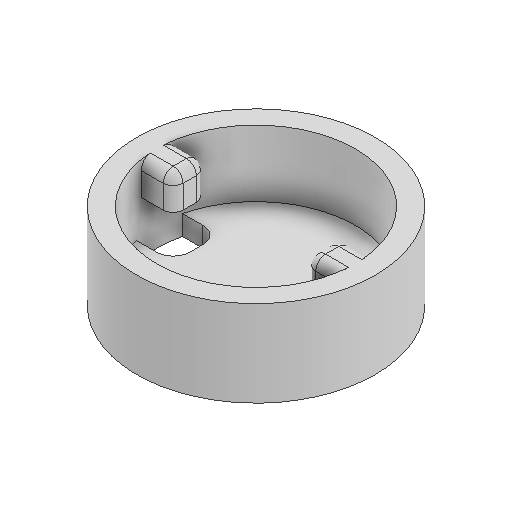
# Autodesk Inventor part: Tapa
Saved by Autodesk Inventor 2025.2 (Build 292293000, 293)
## iProperties
Created: 2025-05-04
Part Number: Tapa
Material: Genérico
Document SubType Name: Modeling
Designer: acer
Density: 1 g/cm^3
Appearance: Valor por defecto
Author: acer
Autodesk Inventor part; units mm, degrees
ref_plane "YZ Plane" through (0, 0, 0) normal (1, 0, 0) x (0, 1, 0)
ref_plane "XZ Plane" through (0, 0, 0) normal (0, 1, 0) x (-1, 0, 0)
ref_plane "XY Plane" through (0, 0, 0) normal (0, 0, 1) x (1, 0, 0)
sketch "Sketch5" plane through (0, 0, 0) normal (0, 1, 0) x (-1, 0, 0)
  circle A0 centre (0, 0) radius 15
  circle A1 centre (0, 0) radius 18
  dimension "d18" = 30
  dimension "d19" = 36
  constraints: 2 centre point, 2 coincident
  measures "d18" diameter of A0
  measures "d19" diameter of A1
extrude "Extrusion4" add sketch "Sketch5" along normal blind 5
sketch "Sketch6" plane through (0, 0, 0) normal (0, -1, 0) x (1, 0, 0)
  circle A0 centre (0, 0) radius 15 projected
  circle A1 centre (0, 0) radius 18 projected
extrude "Extrusion5" add sketch "Sketch6" along normal blind 3 contours A0 | A1
sketch "Sketch7" plane through (0, 5, 0) normal (0, 1, 0) x (1, 0, 0)
  circle A0 centre (0, 0) radius 15 projected
  circle A1 centre (0, 0) radius 18 projected
  line L0 (-17.8255, 2.5) -> (17.8255, 2.5)
  line L1 (-17.8255, -2.5) -> (17.8255, -2.5)
  circle A2 centre (0, 0) radius 10
  line L2 (-10, 2.5) -> (-10, -2.5)
  line L3 (10, 2.5) -> (10, -2.5)
  point P0 (0, 2.5)
  point P1 (-14.7902, 2.5)
  point P2 (14.7902, 2.5)
  point P3 (14.7902, -2.5)
  point P4 (-14.7902, -2.5)
  dimension "d24" = 2.5
  dimension "d25" = 20
  constraints: 8 end point, 4 point on circle, 4 point on line, 1 centre point, 1 coincident, 1 horizontal, 1 midpoint, 1 parallel, 1 perpendicular
  measures "d24" distance of point (0, 2.5) point (0, 0)
  measures "d25" diameter of A2
extrude "Extrusion6" add sketch "Sketch7" along normal blind 5 contours A0 L1 L3 L0 | A0 L0 A1 L1 | A0 L0 A1 | L1 A1 A0 | L0 L2 L1 A0 | A0 L1 A1 L0
fillet "Fillet1" radius 1.5 10 edges at (-10, 7.5, 2.5) (-10, 10, 0) (10, 7.5, 2.5) (10, 10, 0) (10, 7.5, -2.5) (-10, 7.5, -2.5) (12.3951, 10, 2.5) (12.3951, 10, -2.5) (-12.3951, 10, 2.5) (-12.3951, 10, -2.5)
sketch "Sketch8" plane through (0, 0, 0) normal (0, 1, 0) x (1, 0, 0)
  arc A0 (-10, 1) -> (-11.5, 2.5) centre (-11.5, 1) ccw projected
  line L0 (-11.5, 2.5) -> (-14.7902, 2.5) projected
  line L1 (-10, -1) -> (-10, 1) projected
  arc A1 (-11.5, -2.5) -> (-10, -1) centre (-11.5, -1) ccw projected
  line L2 (-14.7902, -2.5) -> (-11.5, -2.5) projected
  line L3 (11.5, -2.5) -> (14.7902, -2.5) projected
  arc A2 (10, -1) -> (11.5, -2.5) centre (11.5, -1) ccw projected
  line L4 (10, 1) -> (10, -1) projected
  arc A3 (11.5, 2.5) -> (10, 1) centre (11.5, 1) ccw projected
  line L5 (14.7902, 2.5) -> (11.5, 2.5) projected
  arc A4 (14.9666, 1) -> (-14.9666, 1) centre (0, 0) ccw projected
  line L6 (-14.7902, -3.5) -> (-11.5, -3.5)
  arc A5 (-11.5, -3.5) -> (-9, -1) centre (-11.5, -1) ccw
  line L7 (-9, -1) -> (-9, 1)
  arc A6 (-9, 1) -> (-11.5, 3.5) centre (-11.5, 1) ccw
  line L8 (-11.5, 3.5) -> (-14.7902, 3.5)
  line L9 (14.7902, -3.5) -> (11.5, -3.5)
  arc A7 (9, -1) -> (11.5, -3.5) centre (11.5, -1) ccw
  line L10 (9, -1) -> (9, 1)
  arc A8 (11.5, 3.5) -> (9, 1) centre (11.5, 1) ccw
  line L11 (11.5, 3.5) -> (14.7902, 3.5)
  circle A9 centre (0, 0) radius 15 projected
  point P0 (14.586, 3.5)
  point P1 (14.586, -3.5)
  point P2 (-14.586, -3.5)
  point P3 (-14.586, 3.5)
  dimension "d29" = 1
  dimension "d30" = 1
  constraints: 12 end point, 8 point on circle, 4 centre point, 8 other
  measures "d29" distance between parallel lines of L2 L6
  measures "d30" radial gap between concentric circles of A3 A8
extrude "Extrusion7" cut sketch "Sketch8" against normal through all contours L1 A1 L2 A9 A4 L0 A0 | A0 L0 A4 L8 A6 L7 A5 L6 A9 L2 A1 L1 | A4 L5 A3 L4 A2 L3 A9 L9 A7 L10 A8 L11 | A4 A9 L3 A2 L4 A3 L5
body "Solid2"
